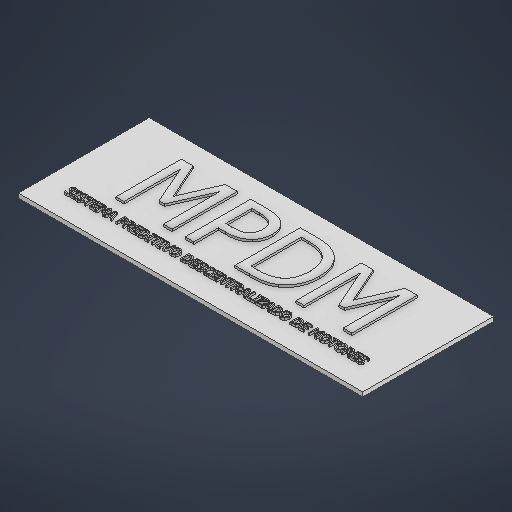
# Autodesk Inventor part: logoR
Saved by Autodesk Inventor 2026.1 (Build 301233020, 233B)
## iProperties
Created: 2025-11-12
Part Number: logoR
Material: Genérico
Document SubType Name: Modeling
Designer: luska
Density: 1 g/cm^3
Appearance: Padrão
Author: luska
## iProperties of the stored document logoR_3DPrint.ipt
Created: 2025-11-12
Part Number: logoR_3DPrint
Material: Genérico
Document SubType Name: Modeling
Designer: luska
Density: 1 g/cm^3
Appearance: Padrão
Author: luska
Autodesk Inventor part; units mm, degrees
ref_plane "YZ Plane" through (0, 0, 0) normal (1, 0, 0) x (0, 1, 0)
ref_plane "XZ Plane" through (0, 0, 0) normal (0, 1, 0) x (-1, 0, 0)
ref_plane "XY Plane" through (0, 0, 0) normal (0, 0, 1) x (1, 0, 0)
sketch "Esboço1" plane through (0, 0, 0) normal (0, 1, 0) x (-1, 0, 0)
  line L0 (65.0365, 6.881) -> (-13.9635, 6.881)
  line L1 (-13.9635, 6.881) -> (-13.9635, -23.119)
  line L2 (-13.9635, -23.119) -> (65.0365, -23.119)
  line L3 (65.0365, -23.119) -> (65.0365, 6.881)
  point P0 (0, 0)
  dimension "d0" = 79
  dimension "d1" = 30
  constraints: 8 end point, 2 parallel, 1 horizontal, 1 perpendicular
  measures "d0" distance between parallel lines of L3 L1
  measures "d1" distance between parallel lines of L2 L0
extrude "Extrusão1" add sketch "Esboço1" along normal blind 1
sketch "Esboço2" plane through (0, 1, 0) normal (0, 1, 0) x (1, 0, 0)
  line L0 (-54.1205, 18.0637) -> (3.0473, 18.0637) construction
  line L1 (3.0473, 18.0637) -> (3.0473, 3.0637) construction
  line L2 (3.0473, 3.0637) -> (-54.1205, 3.0637) construction
  line L3 (-54.1205, 3.0637) -> (-54.1205, 18.0637) construction
  line L4 (-59.7665, 0.1935) -> (8.6922, 0.1935) construction
  line L5 (8.6922, 0.1935) -> (8.6922, -1.8907) construction
  line L6 (8.6922, -1.8907) -> (-59.7665, -1.8907) construction
  line L7 (-59.7665, -1.8907) -> (-59.7665, 0.1935) construction
  line L8 (-65.0365, 23.119) -> (-65.0365, -6.881) projected
  line L9 (13.9635, -6.881) -> (13.9635, 23.119) projected
  line L10 (-39.7404, 3.0637) -> (-41.7339, 3.0637)
  line L11 (-41.7339, 3.0637) -> (-41.7339, 15.9851)
  line L12 (-41.7339, 15.9851) -> (-45.648, 7.1966)
  line L13 (-45.648, 7.1966) -> (-46.8636, 7.1966)
  line L14 (-46.8636, 7.1966) -> (-50.7412, 15.9851)
  line L15 (-50.7412, 15.9851) -> (-50.7412, 3.0637)
  line L16 (-50.7412, 3.0637) -> (-52.601, 3.0637)
  line L17 (-52.601, 3.0637) -> (-52.601, 18.0637)
  line L18 (-52.601, 18.0637) -> (-49.8782, 18.0637)
  line L19 (-49.8782, 18.0637) -> (-46.1342, 9.7128)
  line L20 (-46.1342, 9.7128) -> (-42.5119, 18.0637)
  line L21 (-42.5119, 18.0637) -> (-39.7404, 18.0637)
  line L22 (-39.7404, 18.0637) -> (-39.7404, 3.0637)
  spline S0 degree 2 poles (-27.2201, 13.5418) (-27.2201, 12.5694) (-27.913, 10.819) (-28.5329, 10.2112) knots 0 0 0 1 2 2 2
  spline S1 degree 2 poles (-28.5329, 10.2112) (-29.3109, 9.4454) (-31.4138, 8.6553) (-33.0184, 8.6553) knots 0 0 0 1 2 2 2
  line L23 (-33.0184, 8.6553) -> (-34.708, 8.6553)
  line L24 (-34.708, 8.6553) -> (-34.708, 3.0637)
  line L25 (-34.708, 3.0637) -> (-36.7015, 3.0637)
  line L26 (-36.7015, 3.0637) -> (-36.7015, 18.0637)
  line L27 (-36.7015, 18.0637) -> (-32.9333, 18.0637)
  spline S2 degree 2 poles (-32.9333, 18.0637) (-31.5962, 18.0637) (-29.7242, 17.6261) (-29.007, 17.1277) knots 0 0 0 1 2 2 2
  spline S3 degree 2 poles (-29.007, 17.1277) (-28.1683, 16.5564) (-27.2201, 14.7938) (-27.2201, 13.5418) knots 0 0 0 1 2 2 2
  spline S4 degree 2 poles (-29.2988, 13.481) (-29.2988, 14.259) (-29.8336, 15.4016) (-30.3806, 15.7663) knots 0 0 0 1 2 2 2
  spline S5 degree 2 poles (-30.3806, 15.7663) (-30.8547, 16.0823) (-32.1188, 16.3376) (-33.0548, 16.3376) knots 0 0 0 1 2 2 2
  line L28 (-33.0548, 16.3376) -> (-34.708, 16.3376)
  line L29 (-34.708, 16.3376) -> (-34.708, 10.3571)
  line L30 (-34.708, 10.3571) -> (-33.3466, 10.3571)
  spline S6 degree 2 poles (-33.3466, 10.3571) (-32.131, 10.3571) (-30.6359, 10.746) (-30.1496, 11.2566) knots 0 0 0 1 2 2 2
  spline S7 degree 2 poles (-30.1496, 11.2566) (-29.6999, 11.7063) (-29.2988, 12.7639) (-29.2988, 13.481) knots 0 0 0 1 2 2 2
  spline S8 degree 2 poles (-13.4965, 10.5515) (-13.4965, 8.4972) (-15.1618, 5.1909) (-16.5597, 4.2671) knots 0 0 0 1 2 2 2
  spline S9 degree 2 poles (-16.5597, 4.2671) (-17.7023, 3.5499) (-20.0483, 3.0637) (-21.8717, 3.0637) knots 0 0 0 1 2 2 2
  line L31 (-21.8717, 3.0637) -> (-25.3239, 3.0637)
  line L32 (-25.3239, 3.0637) -> (-25.3239, 18.0637)
  line L33 (-25.3239, 18.0637) -> (-21.9082, 18.0637)
  spline S10 degree 2 poles (-21.9082, 18.0637) (-19.7931, 18.0637) (-17.3863, 17.4316) (-16.5354, 16.8725) knots 0 0 0 1 2 2 2
  spline S11 degree 2 poles (-16.5354, 16.8725) (-15.0889, 15.9122) (-13.4965, 12.7395) (-13.4965, 10.5515) knots 0 0 0 1 2 2 2
  spline S12 degree 2 poles (-15.5751, 10.5759) (-15.5751, 12.3019) (-16.7177, 14.7452) (-17.8482, 15.4381) knots 0 0 0 1 2 2 2
  spline S13 degree 2 poles (-17.8482, 15.4381) (-18.6505, 15.9122) (-20.4616, 16.3376) (-21.8109, 16.3376) knots 0 0 0 1 2 2 2
  line L34 (-21.8109, 16.3376) -> (-23.3304, 16.3376)
  line L35 (-23.3304, 16.3376) -> (-23.3304, 4.7898)
  line L36 (-23.3304, 4.7898) -> (-21.8109, 4.7898)
  spline S14 degree 2 poles (-21.8109, 4.7898) (-20.4859, 4.7898) (-18.4803, 5.2152) (-17.6658, 5.7866) knots 0 0 0 1 2 2 2
  spline S15 degree 2 poles (-17.6658, 5.7866) (-16.6205, 6.4916) (-15.5751, 8.8254) (-15.5751, 10.5759) knots 0 0 0 1 2 2 2
  line L37 (1.5278, 3.0637) -> (-0.4657, 3.0637)
  line L38 (-0.4657, 3.0637) -> (-0.4657, 15.9851)
  line L39 (-0.4657, 15.9851) -> (-4.3798, 7.1966)
  line L40 (-4.3798, 7.1966) -> (-5.5953, 7.1966)
  line L41 (-5.5953, 7.1966) -> (-9.473, 15.9851)
  line L42 (-9.473, 15.9851) -> (-9.473, 3.0637)
  line L43 (-9.473, 3.0637) -> (-11.3328, 3.0637)
  line L44 (-11.3328, 3.0637) -> (-11.3328, 18.0637)
  line L45 (-11.3328, 18.0637) -> (-8.6099, 18.0637)
  line L46 (-8.6099, 18.0637) -> (-4.866, 9.7128)
  line L47 (-4.866, 9.7128) -> (-1.2436, 18.0637)
  line L48 (-1.2436, 18.0637) -> (1.5278, 18.0637)
  line L49 (1.5278, 18.0637) -> (1.5278, 3.0637)
  spline S16 degree 2 poles (-59.0063, -1.8843) (-59.2235, -1.8843) (-59.5282, -1.7935) (-59.6627, -1.7287) knots 0 0 0 1 2 2 2
  line L50 (-59.6627, -1.7287) -> (-59.6627, -1.3948)
  line L51 (-59.6627, -1.3948) -> (-59.6433, -1.3948)
  spline S17 degree 2 poles (-59.6433, -1.3948) (-59.512, -1.518) (-59.1798, -1.6541) (-59.0258, -1.6541) knots 0 0 0 1 2 2 2
  spline S18 degree 2 poles (-59.0258, -1.6541) (-58.8054, -1.6541) (-58.5801, -1.471) (-58.5801, -1.3202) knots 0 0 0 1 2 2 2
  spline S19 degree 2 poles (-58.5801, -1.3202) (-58.5801, -1.2003) (-58.6984, -1.0512) (-58.8264, -1.0139) knots 0 0 0 1 2 2 2
  spline S20 degree 2 poles (-58.8264, -1.0139) (-58.9188, -0.988) (-59.0728, -0.9523) (-59.1879, -0.9232) knots 0 0 0 1 2 2 2
  spline S21 degree 2 poles (-59.1879, -0.9232) (-59.2916, -0.8956) (-59.4553, -0.8129) (-59.5185, -0.7465) knots 0 0 0 1 2 2 2
  spline S22 degree 2 poles (-59.5185, -0.7465) (-59.5801, -0.68) (-59.6482, -0.5018) (-59.6482, -0.3851) knots 0 0 0 1 2 2 2
  spline S23 degree 2 poles (-59.6482, -0.3851) (-59.6482, -0.142) (-59.2689, 0.1871) (-58.9755, 0.1871) knots 0 0 0 1 2 2 2
  spline S24 degree 2 poles (-58.9755, 0.1871) (-58.807, 0.1871) (-58.5088, 0.1206) (-58.3807, 0.0574) knots 0 0 0 1 2 2 2
  line L52 (-58.3807, 0.0574) -> (-58.3807, -0.2603)
  line L53 (-58.3807, -0.2603) -> (-58.4002, -0.2603)
  spline S25 degree 2 poles (-58.4002, -0.2603) (-58.4958, -0.1728) (-58.794, -0.0431) (-58.9577, -0.0431) knots 0 0 0 1 2 2 2
  spline S26 degree 2 poles (-58.9577, -0.0431) (-59.1425, -0.0431) (-59.371, -0.2165) (-59.371, -0.3575) knots 0 0 0 1 2 2 2
  spline S27 degree 2 poles (-59.371, -0.3575) (-59.371, -0.4839) (-59.2365, -0.6347) (-59.1101, -0.6687) knots 0 0 0 1 2 2 2
  spline S28 degree 2 poles (-59.1101, -0.6687) (-59.0258, -0.6914) (-58.7811, -0.7497) (-58.7, -0.774) knots 0 0 0 1 2 2 2
  spline S29 degree 2 poles (-58.7, -0.774) (-58.4942, -0.8373) (-58.3029, -1.0917) (-58.3029, -1.2781) knots 0 0 0 1 2 2 2
  spline S30 degree 2 poles (-58.3029, -1.2781) (-58.3029, -1.3964) (-58.3986, -1.6233) (-58.4845, -1.7027) knots 0 0 0 1 2 2 2
  spline S31 degree 2 poles (-58.4845, -1.7027) (-58.5801, -1.7903) (-58.8232, -1.8843) (-59.0063, -1.8843) knots 0 0 0 1 2 2 2
  line L54 (-57.3353, -1.8486) -> (-58.1101, -1.8486)
  line L55 (-58.1101, -1.8486) -> (-58.1101, -1.6444)
  line L56 (-58.1101, -1.6444) -> (-57.8556, -1.6444)
  line L57 (-57.8556, -1.6444) -> (-57.8556, -0.0528)
  line L58 (-57.8556, -0.0528) -> (-58.1101, -0.0528)
  line L59 (-58.1101, -0.0528) -> (-58.1101, 0.1514)
  line L60 (-58.1101, 0.1514) -> (-57.3353, 0.1514)
  line L61 (-57.3353, 0.1514) -> (-57.3353, -0.0528)
  line L62 (-57.3353, -0.0528) -> (-57.5898, -0.0528)
  line L63 (-57.5898, -0.0528) -> (-57.5898, -1.6444)
  line L64 (-57.5898, -1.6444) -> (-57.3353, -1.6444)
  line L65 (-57.3353, -1.6444) -> (-57.3353, -1.8486)
  spline S32 degree 2 poles (-56.4488, -1.8843) (-56.666, -1.8843) (-56.9707, -1.7935) (-57.1052, -1.7287) knots 0 0 0 1 2 2 2
  line L66 (-57.1052, -1.7287) -> (-57.1052, -1.3948)
  line L67 (-57.1052, -1.3948) -> (-57.0858, -1.3948)
  spline S33 degree 2 poles (-57.0858, -1.3948) (-56.9545, -1.518) (-56.6222, -1.6541) (-56.4683, -1.6541) knots 0 0 0 1 2 2 2
  spline S34 degree 2 poles (-56.4683, -1.6541) (-56.2478, -1.6541) (-56.0225, -1.471) (-56.0225, -1.3202) knots 0 0 0 1 2 2 2
  spline S35 degree 2 poles (-56.0225, -1.3202) (-56.0225, -1.2003) (-56.1409, -1.0512) (-56.2689, -1.0139) knots 0 0 0 1 2 2 2
  spline S36 degree 2 poles (-56.2689, -1.0139) (-56.3613, -0.988) (-56.5153, -0.9523) (-56.6303, -0.9232) knots 0 0 0 1 2 2 2
  spline S37 degree 2 poles (-56.6303, -0.9232) (-56.7341, -0.8956) (-56.8977, -0.8129) (-56.961, -0.7465) knots 0 0 0 1 2 2 2
  spline S38 degree 2 poles (-56.961, -0.7465) (-57.0225, -0.68) (-57.0906, -0.5018) (-57.0906, -0.3851) knots 0 0 0 1 2 2 2
  spline S39 degree 2 poles (-57.0906, -0.3851) (-57.0906, -0.142) (-56.7114, 0.1871) (-56.418, 0.1871) knots 0 0 0 1 2 2 2
  spline S40 degree 2 poles (-56.418, 0.1871) (-56.2495, 0.1871) (-55.9512, 0.1206) (-55.8232, 0.0574) knots 0 0 0 1 2 2 2
  line L68 (-55.8232, 0.0574) -> (-55.8232, -0.2603)
  line L69 (-55.8232, -0.2603) -> (-55.8426, -0.2603)
  spline S41 degree 2 poles (-55.8426, -0.2603) (-55.9383, -0.1728) (-56.2365, -0.0431) (-56.4002, -0.0431) knots 0 0 0 1 2 2 2
  spline S42 degree 2 poles (-56.4002, -0.0431) (-56.5849, -0.0431) (-56.8135, -0.2165) (-56.8135, -0.3575) knots 0 0 0 1 2 2 2
  spline S43 degree 2 poles (-56.8135, -0.3575) (-56.8135, -0.4839) (-56.6789, -0.6347) (-56.5525, -0.6687) knots 0 0 0 1 2 2 2
  spline S44 degree 2 poles (-56.5525, -0.6687) (-56.4683, -0.6914) (-56.2235, -0.7497) (-56.1425, -0.774) knots 0 0 0 1 2 2 2
  spline S45 degree 2 poles (-56.1425, -0.774) (-55.9366, -0.8373) (-55.7454, -1.0917) (-55.7454, -1.2781) knots 0 0 0 1 2 2 2
  spline S46 degree 2 poles (-55.7454, -1.2781) (-55.7454, -1.3964) (-55.841, -1.6233) (-55.9269, -1.7027) knots 0 0 0 1 2 2 2
  spline S47 degree 2 poles (-55.9269, -1.7027) (-56.0225, -1.7903) (-56.2657, -1.8843) (-56.4488, -1.8843) knots 0 0 0 1 2 2 2
  line L70 (-55.008, -1.8486) -> (-55.008, -0.0852)
  line L71 (-55.008, -0.0852) -> (-55.6789, -0.0852)
  line L72 (-55.6789, -0.0852) -> (-55.6789, 0.1514)
  line L73 (-55.6789, 0.1514) -> (-54.0712, 0.1514)
  line L74 (-54.0712, 0.1514) -> (-54.0712, -0.0852)
  line L75 (-54.0712, -0.0852) -> (-54.7422, -0.0852)
  line L76 (-54.7422, -0.0852) -> (-54.7422, -1.8486)
  line L77 (-54.7422, -1.8486) -> (-55.008, -1.8486)
  line L78 (-53.8686, -1.8486) -> (-53.8686, 0.1514)
  line L79 (-53.8686, 0.1514) -> (-52.6174, 0.1514)
  line L80 (-52.6174, 0.1514) -> (-52.6174, -0.0852)
  line L81 (-52.6174, -0.0852) -> (-53.6028, -0.0852)
  line L82 (-53.6028, -0.0852) -> (-53.6028, -0.633)
  line L83 (-53.6028, -0.633) -> (-52.6838, -0.633)
  line L84 (-52.6838, -0.633) -> (-52.6838, -0.8697)
  line L85 (-52.6838, -0.8697) -> (-53.6028, -0.8697)
  line L86 (-53.6028, -0.8697) -> (-53.6028, -1.612)
  line L87 (-53.6028, -1.612) -> (-52.6174, -1.612)
  line L88 (-52.6174, -1.612) -> (-52.6174, -1.8486)
  line L89 (-52.6174, -1.8486) -> (-53.8686, -1.8486)
  line L90 (-50.6109, -1.8486) -> (-50.8767, -1.8486)
  line L91 (-50.8767, -1.8486) -> (-50.8767, -0.1258)
  line L92 (-50.8767, -0.1258) -> (-51.3986, -1.2976)
  line L93 (-51.3986, -1.2976) -> (-51.5606, -1.2976)
  line L94 (-51.5606, -1.2976) -> (-52.0777, -0.1258)
  line L95 (-52.0777, -0.1258) -> (-52.0777, -1.8486)
  line L96 (-52.0777, -1.8486) -> (-52.3256, -1.8486)
  line L97 (-52.3256, -1.8486) -> (-52.3256, 0.1514)
  line L98 (-52.3256, 0.1514) -> (-51.9626, 0.1514)
  line L99 (-51.9626, 0.1514) -> (-51.4634, -0.9621)
  line L100 (-51.4634, -0.9621) -> (-50.9804, 0.1514)
  line L101 (-50.9804, 0.1514) -> (-50.6109, 0.1514)
  line L102 (-50.6109, 0.1514) -> (-50.6109, -1.8486)
  line L103 (-50.4212, -1.8486) -> (-49.747, 0.1514)
  line L104 (-49.747, 0.1514) -> (-49.4196, 0.1514)
  line L105 (-49.4196, 0.1514) -> (-48.7454, -1.8486)
  line L106 (-48.7454, -1.8486) -> (-49.0258, -1.8486)
  line L107 (-49.0258, -1.8486) -> (-49.2073, -1.2894)
  line L108 (-49.2073, -1.2894) -> (-49.9707, -1.2894)
  line L109 (-49.9707, -1.2894) -> (-50.1522, -1.8486)
  line L110 (-50.1522, -1.8486) -> (-50.4212, -1.8486)
  line L111 (-49.2802, -1.0625) -> (-49.5898, -0.1209)
  line L112 (-49.5898, -0.1209) -> (-49.8977, -1.0625)
  line L113 (-49.8977, -1.0625) -> (-49.2802, -1.0625)
  spline S48 degree 2 poles (-46.4326, -0.4515) (-46.4326, -0.5812) (-46.525, -0.8146) (-46.6076, -0.8956) knots 0 0 0 1 2 2 2
  spline S49 degree 2 poles (-46.6076, -0.8956) (-46.7114, -0.9977) (-46.9918, -1.1031) (-47.2057, -1.1031) knots 0 0 0 1 2 2 2
  line L114 (-47.2057, -1.1031) -> (-47.431, -1.1031)
  line L115 (-47.431, -1.1031) -> (-47.431, -1.8486)
  line L116 (-47.431, -1.8486) -> (-47.6968, -1.8486)
  line L117 (-47.6968, -1.8486) -> (-47.6968, 0.1514)
  line L118 (-47.6968, 0.1514) -> (-47.1943, 0.1514)
  spline S50 degree 2 poles (-47.1943, 0.1514) (-47.0161, 0.1514) (-46.7665, 0.093) (-46.6708, 0.0266) knots 0 0 0 1 2 2 2
  spline S51 degree 2 poles (-46.6708, 0.0266) (-46.559, -0.0496) (-46.4326, -0.2846) (-46.4326, -0.4515) knots 0 0 0 1 2 2 2
  spline S52 degree 2 poles (-46.7097, -0.4596) (-46.7097, -0.3559) (-46.7811, -0.2035) (-46.854, -0.1549) knots 0 0 0 1 2 2 2
  spline S53 degree 2 poles (-46.854, -0.1549) (-46.9172, -0.1128) (-47.0858, -0.0787) (-47.2106, -0.0787) knots 0 0 0 1 2 2 2
  line L119 (-47.2106, -0.0787) -> (-47.431, -0.0787)
  line L120 (-47.431, -0.0787) -> (-47.431, -0.8762)
  line L121 (-47.431, -0.8762) -> (-47.2495, -0.8762)
  spline S54 degree 2 poles (-47.2495, -0.8762) (-47.0874, -0.8762) (-46.888, -0.8243) (-46.8232, -0.7562) knots 0 0 0 1 2 2 2
  spline S55 degree 2 poles (-46.8232, -0.7562) (-46.7632, -0.6963) (-46.7097, -0.5552) (-46.7097, -0.4596) knots 0 0 0 1 2 2 2
  line L122 (-44.6319, -1.8486) -> (-44.9772, -1.8486)
  line L123 (-44.9772, -1.8486) -> (-45.6093, -1.0528)
  line L124 (-45.6093, -1.0528) -> (-45.914, -1.0528)
  line L125 (-45.914, -1.0528) -> (-45.914, -1.8486)
  line L126 (-45.914, -1.8486) -> (-46.1798, -1.8486)
  line L127 (-46.1798, -1.8486) -> (-46.1798, 0.1514)
  line L128 (-46.1798, 0.1514) -> (-45.6644, 0.1514)
  spline S56 degree 2 poles (-45.6644, 0.1514) (-45.4926, 0.1514) (-45.2608, 0.1141) (-45.1554, 0.046) knots 0 0 0 1 2 2 2
  spline S57 degree 2 poles (-45.1554, 0.046) (-45.0501, -0.022) (-44.9285, -0.2343) (-44.9285, -0.3916) knots 0 0 0 1 2 2 2
  spline S58 degree 2 poles (-44.9285, -0.3916) (-44.9285, -0.6104) (-45.1522, -0.907) (-45.3435, -0.9783) knots 0 0 0 1 2 2 2
  line L129 (-45.3435, -0.9783) -> (-44.6319, -1.8486)
  spline S59 degree 2 poles (-45.2057, -0.4126) (-45.2057, -0.3251) (-45.2673, -0.1906) (-45.3321, -0.1468) knots 0 0 0 1 2 2 2
  spline S60 degree 2 poles (-45.3321, -0.1468) (-45.3888, -0.1095) (-45.5396, -0.0787) (-45.6498, -0.0787) knots 0 0 0 1 2 2 2
  line L130 (-45.6498, -0.0787) -> (-45.914, -0.0787)
  line L131 (-45.914, -0.0787) -> (-45.914, -0.8308)
  line L132 (-45.914, -0.8308) -> (-45.6806, -0.8308)
  spline S61 degree 2 poles (-45.6806, -0.8308) (-45.5655, -0.8308) (-45.3824, -0.7903) (-45.3191, -0.727) knots 0 0 0 1 2 2 2
  spline S62 degree 2 poles (-45.3191, -0.727) (-45.2608, -0.6719) (-45.2057, -0.5164) (-45.2057, -0.4126) knots 0 0 0 1 2 2 2
  line L133 (-44.4731, -1.8486) -> (-44.4731, 0.1514)
  line L134 (-44.4731, 0.1514) -> (-43.2219, 0.1514)
  line L135 (-43.2219, 0.1514) -> (-43.2219, -0.0852)
  line L136 (-43.2219, -0.0852) -> (-44.2073, -0.0852)
  line L137 (-44.2073, -0.0852) -> (-44.2073, -0.633)
  line L138 (-44.2073, -0.633) -> (-43.2883, -0.633)
  line L139 (-43.2883, -0.633) -> (-43.2883, -0.8697)
  line L140 (-43.2883, -0.8697) -> (-44.2073, -0.8697)
  line L141 (-44.2073, -0.8697) -> (-44.2073, -1.612)
  line L142 (-44.2073, -1.612) -> (-43.2219, -1.612)
  line L143 (-43.2219, -1.612) -> (-43.2219, -1.8486)
  line L144 (-43.2219, -1.8486) -> (-44.4731, -1.8486)
  spline S63 degree 2 poles (-41.3532, -0.8502) (-41.3532, -1.1241) (-41.5752, -1.565) (-41.7616, -1.6881) knots 0 0 0 1 2 2 2
  spline S64 degree 2 poles (-41.7616, -1.6881) (-41.914, -1.7838) (-42.2268, -1.8486) (-42.4699, -1.8486) knots 0 0 0 1 2 2 2
  line L145 (-42.4699, -1.8486) -> (-42.9302, -1.8486)
  line L146 (-42.9302, -1.8486) -> (-42.9302, 0.1514)
  line L147 (-42.9302, 0.1514) -> (-42.4747, 0.1514)
  spline S65 degree 2 poles (-42.4747, 0.1514) (-42.1927, 0.1514) (-41.8718, 0.0671) (-41.7584, -0.0074) knots 0 0 0 1 2 2 2
  spline S66 degree 2 poles (-41.7584, -0.0074) (-41.5655, -0.1355) (-41.3532, -0.5585) (-41.3532, -0.8502) knots 0 0 0 1 2 2 2
  spline S67 degree 2 poles (-41.6303, -0.847) (-41.6303, -0.6168) (-41.7827, -0.2911) (-41.9334, -0.1987) knots 0 0 0 1 2 2 2
  spline S68 degree 2 poles (-41.9334, -0.1987) (-42.0404, -0.1355) (-42.2819, -0.0787) (-42.4618, -0.0787) knots 0 0 0 1 2 2 2
  line L148 (-42.4618, -0.0787) -> (-42.6644, -0.0787)
  line L149 (-42.6644, -0.0787) -> (-42.6644, -1.6185)
  line L150 (-42.6644, -1.6185) -> (-42.4618, -1.6185)
  spline S69 degree 2 poles (-42.4618, -1.6185) (-42.2851, -1.6185) (-42.0177, -1.5617) (-41.9091, -1.4856) knots 0 0 0 1 2 2 2
  spline S70 degree 2 poles (-41.9091, -1.4856) (-41.7697, -1.3916) (-41.6303, -1.0804) (-41.6303, -0.847) knots 0 0 0 1 2 2 2
  line L151 (-40.3678, -1.8486) -> (-41.1425, -1.8486)
  line L152 (-41.1425, -1.8486) -> (-41.1425, -1.6444)
  line L153 (-41.1425, -1.6444) -> (-40.888, -1.6444)
  line L154 (-40.888, -1.6444) -> (-40.888, -0.0528)
  line L155 (-40.888, -0.0528) -> (-41.1425, -0.0528)
  line L156 (-41.1425, -0.0528) -> (-41.1425, 0.1514)
  line L157 (-41.1425, 0.1514) -> (-40.3678, 0.1514)
  line L158 (-40.3678, 0.1514) -> (-40.3678, -0.0528)
  line L159 (-40.3678, -0.0528) -> (-40.6222, -0.0528)
  line L160 (-40.6222, -0.0528) -> (-40.6222, -1.6444)
  line L161 (-40.6222, -1.6444) -> (-40.3678, -1.6444)
  line L162 (-40.3678, -1.6444) -> (-40.3678, -1.8486)
  line L163 (-39.572, -1.8486) -> (-39.572, -0.0852)
  line L164 (-39.572, -0.0852) -> (-40.243, -0.0852)
  line L165 (-40.243, -0.0852) -> (-40.243, 0.1514)
  line L166 (-40.243, 0.1514) -> (-38.6352, 0.1514)
  line L167 (-38.6352, 0.1514) -> (-38.6352, -0.0852)
  line L168 (-38.6352, -0.0852) -> (-39.3062, -0.0852)
  line L169 (-39.3062, -0.0852) -> (-39.3062, -1.8486)
  line L170 (-39.3062, -1.8486) -> (-39.572, -1.8486)
  line L171 (-37.7357, -1.8486) -> (-38.5104, -1.8486)
  line L172 (-38.5104, -1.8486) -> (-38.5104, -1.6444)
  line L173 (-38.5104, -1.6444) -> (-38.2559, -1.6444)
  line L174 (-38.2559, -1.6444) -> (-38.2559, -0.0528)
  line L175 (-38.2559, -0.0528) -> (-38.5104, -0.0528)
  line L176 (-38.5104, -0.0528) -> (-38.5104, 0.1514)
  line L177 (-38.5104, 0.1514) -> (-37.7357, 0.1514)
  line L178 (-37.7357, 0.1514) -> (-37.7357, -0.0528)
  line L179 (-37.7357, -0.0528) -> (-37.9901, -0.0528)
  line L180 (-37.9901, -0.0528) -> (-37.9901, -1.6444)
  line L181 (-37.9901, -1.6444) -> (-37.7357, -1.6444)
  line L182 (-37.7357, -1.6444) -> (-37.7357, -1.8486)
  line L183 (-35.9561, 0.1514) -> (-36.6449, -1.8486)
  line L184 (-36.6449, -1.8486) -> (-36.9318, -1.8486)
  line L185 (-36.9318, -1.8486) -> (-37.6206, 0.1514)
  line L186 (-37.6206, 0.1514) -> (-37.3353, 0.1514)
  line L187 (-37.3353, 0.1514) -> (-36.7811, -1.5099)
  line L188 (-36.7811, -1.5099) -> (-36.2268, 0.1514)
  line L189 (-36.2268, 0.1514) -> (-35.9561, 0.1514)
  spline S71 degree 2 poles (-34.3499, -0.0771) (-34.2365, -0.21) (-34.1101, -0.599) (-34.1101, -0.8486) knots 0 0 0 1 2 2 2
  spline S72 degree 2 poles (-34.1101, -0.8486) (-34.1101, -1.0917) (-34.2332, -1.4856) (-34.3499, -1.6185) knots 0 0 0 1 2 2 2
  spline S73 degree 2 poles (-34.3499, -1.6185) (-34.4731, -1.7578) (-34.7989, -1.8907) (-34.995, -1.8907) knots 0 0 0 1 2 2 2
  spline S74 degree 2 poles (-34.995, -1.8907) (-35.1976, -1.8907) (-35.5217, -1.753) (-35.64, -1.6185) knots 0 0 0 1 2 2 2
  spline S75 degree 2 poles (-35.64, -1.6185) (-35.7551, -1.4856) (-35.8783, -1.095) (-35.8783, -0.8486) knots 0 0 0 1 2 2 2
  spline S76 degree 2 poles (-35.8783, -0.8486) (-35.8783, -0.5974) (-35.7535, -0.2149) (-35.6384, -0.0771) knots 0 0 0 1 2 2 2
  spline S77 degree 2 poles (-35.6384, -0.0771) (-35.5217, 0.0558) (-35.196, 0.1935) (-34.995, 0.1935) knots 0 0 0 1 2 2 2
  spline S78 degree 2 poles (-34.995, 0.1935) (-34.7908, 0.1935) (-34.4634, 0.0509) (-34.3499, -0.0771) knots 0 0 0 1 2 2 2
  spline S79 degree 2 poles (-34.3872, -0.8486) (-34.3872, -0.6509) (-34.4731, -0.3446) (-34.5509, -0.2441) knots 0 0 0 1 2 2 2
  spline S80 degree 2 poles (-34.5509, -0.2441) (-34.6303, -0.1403) (-34.854, -0.0366) (-34.9934, -0.0366) knots 0 0 0 1 2 2 2
  spline S81 degree 2 poles (-34.9934, -0.0366) (-35.1376, -0.0366) (-35.3548, -0.1371) (-35.4375, -0.2441) knots 0 0 0 1 2 2 2
  spline S82 degree 2 poles (-35.4375, -0.2441) (-35.5169, -0.3462) (-35.6012, -0.6541) (-35.6012, -0.8486) knots 0 0 0 1 2 2 2
  spline S83 degree 2 poles (-35.6012, -0.8486) (-35.6012, -1.2424) (-35.2705, -1.6606) (-34.9934, -1.6606) knots 0 0 0 1 2 2 2
  spline S84 degree 2 poles (-34.9934, -1.6606) (-34.7162, -1.6606) (-34.3872, -1.2424) (-34.3872, -0.8486) knots 0 0 0 1 2 2 2
  spline S85 degree 2 poles (-31.3824, -0.8502) (-31.3824, -1.1241) (-31.6044, -1.565) (-31.7908, -1.6881) knots 0 0 0 1 2 2 2
  spline S86 degree 2 poles (-31.7908, -1.6881) (-31.9431, -1.7838) (-32.2559, -1.8486) (-32.499, -1.8486) knots 0 0 0 1 2 2 2
  line L190 (-32.499, -1.8486) -> (-32.9593, -1.8486)
  line L191 (-32.9593, -1.8486) -> (-32.9593, 0.1514)
  line L192 (-32.9593, 0.1514) -> (-32.5039, 0.1514)
  spline S87 degree 2 poles (-32.5039, 0.1514) (-32.2219, 0.1514) (-31.901, 0.0671) (-31.7875, -0.0074) knots 0 0 0 1 2 2 2
  spline S88 degree 2 poles (-31.7875, -0.0074) (-31.5947, -0.1355) (-31.3824, -0.5585) (-31.3824, -0.8502) knots 0 0 0 1 2 2 2
  spline S89 degree 2 poles (-31.6595, -0.847) (-31.6595, -0.6168) (-31.8118, -0.2911) (-31.9626, -0.1987) knots 0 0 0 1 2 2 2
  spline S90 degree 2 poles (-31.9626, -0.1987) (-32.0695, -0.1355) (-32.311, -0.0787) (-32.4909, -0.0787) knots 0 0 0 1 2 2 2
  line L193 (-32.4909, -0.0787) -> (-32.6935, -0.0787)
  line L194 (-32.6935, -0.0787) -> (-32.6935, -1.6185)
  line L195 (-32.6935, -1.6185) -> (-32.4909, -1.6185)
  spline S91 degree 2 poles (-32.4909, -1.6185) (-32.3143, -1.6185) (-32.0469, -1.5617) (-31.9383, -1.4856) knots 0 0 0 1 2 2 2
  spline S92 degree 2 poles (-31.9383, -1.4856) (-31.7989, -1.3916) (-31.6595, -1.0804) (-31.6595, -0.847) knots 0 0 0 1 2 2 2
  line L196 (-31.0939, -1.8486) -> (-31.0939, 0.1514)
  line L197 (-31.0939, 0.1514) -> (-29.8426, 0.1514)
  line L198 (-29.8426, 0.1514) -> (-29.8426, -0.0852)
  line L199 (-29.8426, -0.0852) -> (-30.8281, -0.0852)
  line L200 (-30.8281, -0.0852) -> (-30.8281, -0.633)
  line L201 (-30.8281, -0.633) -> (-29.9091, -0.633)
  line L202 (-29.9091, -0.633) -> (-29.9091, -0.8697)
  line L203 (-29.9091, -0.8697) -> (-30.8281, -0.8697)
  line L204 (-30.8281, -0.8697) -> (-30.8281, -1.612)
  line L205 (-30.8281, -1.612) -> (-29.8426, -1.612)
  line L206 (-29.8426, -1.612) -> (-29.8426, -1.8486)
  line L207 (-29.8426, -1.8486) -> (-31.0939, -1.8486)
  spline S93 degree 2 poles (-28.9934, -1.8843) (-29.2106, -1.8843) (-29.5153, -1.7935) (-29.6498, -1.7287) knots 0 0 0 1 2 2 2
  line L208 (-29.6498, -1.7287) -> (-29.6498, -1.3948)
  line L209 (-29.6498, -1.3948) -> (-29.6303, -1.3948)
  spline S94 degree 2 poles (-29.6303, -1.3948) (-29.499, -1.518) (-29.1668, -1.6541) (-29.0128, -1.6541) knots 0 0 0 1 2 2 2
  spline S95 degree 2 poles (-29.0128, -1.6541) (-28.7924, -1.6541) (-28.5671, -1.471) (-28.5671, -1.3202) knots 0 0 0 1 2 2 2
  spline S96 degree 2 poles (-28.5671, -1.3202) (-28.5671, -1.2003) (-28.6854, -1.0512) (-28.8135, -1.0139) knots 0 0 0 1 2 2 2
  spline S97 degree 2 poles (-28.8135, -1.0139) (-28.9059, -0.988) (-29.0598, -0.9523) (-29.1749, -0.9232) knots 0 0 0 1 2 2 2
  spline S98 degree 2 poles (-29.1749, -0.9232) (-29.2786, -0.8956) (-29.4423, -0.8129) (-29.5055, -0.7465) knots 0 0 0 1 2 2 2
  spline S99 degree 2 poles (-29.5055, -0.7465) (-29.5671, -0.68) (-29.6352, -0.5018) (-29.6352, -0.3851) knots 0 0 0 1 2 2 2
  spline S100 degree 2 poles (-29.6352, -0.3851) (-29.6352, -0.142) (-29.2559, 0.1871) (-28.9626, 0.1871) knots 0 0 0 1 2 2 2
  spline S101 degree 2 poles (-28.9626, 0.1871) (-28.794, 0.1871) (-28.4958, 0.1206) (-28.3678, 0.0574) knots 0 0 0 1 2 2 2
  line L210 (-28.3678, 0.0574) -> (-28.3678, -0.2603)
  line L211 (-28.3678, -0.2603) -> (-28.3872, -0.2603)
  spline S102 degree 2 poles (-28.3872, -0.2603) (-28.4828, -0.1728) (-28.7811, -0.0431) (-28.9447, -0.0431) knots 0 0 0 1 2 2 2
  spline S103 degree 2 poles (-28.9447, -0.0431) (-29.1295, -0.0431) (-29.358, -0.2165) (-29.358, -0.3575) knots 0 0 0 1 2 2 2
  spline S104 degree 2 poles (-29.358, -0.3575) (-29.358, -0.4839) (-29.2235, -0.6347) (-29.0971, -0.6687) knots 0 0 0 1 2 2 2
  spline S105 degree 2 poles (-29.0971, -0.6687) (-29.0128, -0.6914) (-28.7681, -0.7497) (-28.6871, -0.774) knots 0 0 0 1 2 2 2
  spline S106 degree 2 poles (-28.6871, -0.774) (-28.4812, -0.8373) (-28.29, -1.0917) (-28.29, -1.2781) knots 0 0 0 1 2 2 2
  spline S107 degree 2 poles (-28.29, -1.2781) (-28.29, -1.3964) (-28.3856, -1.6233) (-28.4715, -1.7027) knots 0 0 0 1 2 2 2
  spline S108 degree 2 poles (-28.4715, -1.7027) (-28.5671, -1.7903) (-28.8102, -1.8843) (-28.9934, -1.8843) knots 0 0 0 1 2 2 2
  spline S109 degree 2 poles (-27.2381, -1.8843) (-27.4326, -1.8843) (-27.7616, -1.753) (-27.8815, -1.6217) knots 0 0 0 1 2 2 2
  spline S110 degree 2 poles (-27.8815, -1.6217) (-28.0015, -1.492) (-28.1328, -1.1031) (-28.1328, -0.8502) knots 0 0 0 1 2 2 2
  spline S111 degree 2 poles (-28.1328, -0.8502) (-28.1328, -0.599) (-28.0047, -0.2262) (-27.8832, -0.0885) knots 0 0 0 1 2 2 2
  spline S112 degree 2 poles (-27.8832, -0.0885) (-27.7632, 0.046) (-27.4358, 0.1871) (-27.2332, 0.1871) knots 0 0 0 1 2 2 2
  spline S113 degree 2 poles (-27.2332, 0.1871) (-27.1328, 0.1871) (-26.9561, 0.1579) (-26.8815, 0.1352) knots 0 0 0 1 2 2 2
  spline S114 degree 2 poles (-26.8815, 0.1352) (-26.8167, 0.1141) (-26.6822, 0.0542) (-26.6157, 0.0185) knots 0 0 0 1 2 2 2
  line L212 (-26.6157, 0.0185) -> (-26.6157, -0.3024)
  line L213 (-26.6157, -0.3024) -> (-26.6368, -0.3024)
  spline S115 degree 2 poles (-26.6368, -0.3024) (-26.6725, -0.27) (-26.7827, -0.1792) (-26.8621, -0.1355) knots 0 0 0 1 2 2 2
  spline S116 degree 2 poles (-26.8621, -0.1355) (-26.9383, -0.0933) (-27.1182, -0.0399) (-27.2349, -0.0399) knots 0 0 0 1 2 2 2
  spline S117 degree 2 poles (-27.2349, -0.0399) (-27.3629, -0.0399) (-27.5914, -0.1452) (-27.6773, -0.2457) knots 0 0 0 1 2 2 2
  spline S118 degree 2 poles (-27.6773, -0.2457) (-27.7616, -0.3478) (-27.8556, -0.6574) (-27.8556, -0.8502) knots 0 0 0 1 2 2 2
  spline S119 degree 2 poles (-27.8556, -0.8502) (-27.8556, -1.0561) (-27.7567, -1.3527) (-27.6708, -1.4548) knots 0 0 0 1 2 2 2
  spline S120 degree 2 poles (-27.6708, -1.4548) (-27.5866, -1.5536) (-27.3613, -1.6541) (-27.2349, -1.6541) knots 0 0 0 1 2 2 2
  spline S121 degree 2 poles (-27.2349, -1.6541) (-27.1198, -1.6541) (-26.9237, -1.5974) (-26.8475, -1.5552) knots 0 0 0 1 2 2 2
  spline S122 degree 2 poles (-26.8475, -1.5552) (-26.7746, -1.5131) (-26.666, -1.4256) (-26.6352, -1.3948) knots 0 0 0 1 2 2 2
  line L214 (-26.6352, -1.3948) -> (-26.6157, -1.3948)
  line L215 (-26.6157, -1.3948) -> (-26.6157, -1.7125)
  spline S123 degree 2 poles (-26.6157, -1.7125) (-26.6822, -1.7433) (-26.7989, -1.8) (-26.8815, -1.8259) knots 0 0 0 1 2 2 2
  spline S124 degree 2 poles (-26.8815, -1.8259) (-26.9691, -1.8551) (-27.1182, -1.8843) (-27.2381, -1.8843) knots 0 0 0 1 2 2 2
  line L216 (-26.3678, -1.8486) -> (-26.3678, 0.1514)
  line L217 (-26.3678, 0.1514) -> (-25.1165, 0.1514)
  line L218 (-25.1165, 0.1514) -> (-25.1165, -0.0852)
  line L219 (-25.1165, -0.0852) -> (-26.102, -0.0852)
  line L220 (-26.102, -0.0852) -> (-26.102, -0.633)
  line L221 (-26.102, -0.633) -> (-25.183, -0.633)
  line L222 (-25.183, -0.633) -> (-25.183, -0.8697)
  line L223 (-25.183, -0.8697) -> (-26.102, -0.8697)
  line L224 (-26.102, -0.8697) -> (-26.102, -1.612)
  line L225 (-26.102, -1.612) -> (-25.1165, -1.612)
  line L226 (-25.1165, -1.612) -> (-25.1165, -1.8486)
  line L227 (-25.1165, -1.8486) -> (-26.3678, -1.8486)
  line L228 (-23.3937, -1.8486) -> (-23.6919, -1.8486)
  line L229 (-23.6919, -1.8486) -> (-24.5768, -0.1241)
  line L230 (-24.5768, -0.1241) -> (-24.5768, -1.8486)
  line L231 (-24.5768, -1.8486) -> (-24.8248, -1.8486)
  line L232 (-24.8248, -1.8486) -> (-24.8248, 0.1514)
  line L233 (-24.8248, 0.1514) -> (-24.4472, 0.1514)
  line L234 (-24.4472, 0.1514) -> (-23.6417, -1.4321)
  line L235 (-23.6417, -1.4321) -> (-23.6417, 0.1514)
  line L236 (-23.6417, 0.1514) -> (-23.3937, 0.1514)
  line L237 (-23.3937, 0.1514) -> (-23.3937, -1.8486)
  line L238 (-22.5217, -1.8486) -> (-22.5217, -0.0852)
  line L239 (-22.5217, -0.0852) -> (-23.1927, -0.0852)
  line L240 (-23.1927, -0.0852) -> (-23.1927, 0.1514)
  line L241 (-23.1927, 0.1514) -> (-21.5849, 0.1514)
  line L242 (-21.5849, 0.1514) -> (-21.5849, -0.0852)
  line L243 (-21.5849, -0.0852) -> (-22.2559, -0.0852)
  line L244 (-22.2559, -0.0852) -> (-22.2559, -1.8486)
  line L245 (-22.2559, -1.8486) -> (-22.5217, -1.8486)
  line L246 (-19.8345, -1.8486) -> (-20.1798, -1.8486)
  line L247 (-20.1798, -1.8486) -> (-20.8118, -1.0528)
  line L248 (-20.8118, -1.0528) -> (-21.1165, -1.0528)
  line L249 (-21.1165, -1.0528) -> (-21.1165, -1.8486)
  line L250 (-21.1165, -1.8486) -> (-21.3824, -1.8486)
  line L251 (-21.3824, -1.8486) -> (-21.3824, 0.1514)
  line L252 (-21.3824, 0.1514) -> (-20.867, 0.1514)
  spline S125 degree 2 poles (-20.867, 0.1514) (-20.6952, 0.1514) (-20.4634, 0.1141) (-20.358, 0.046) knots 0 0 0 1 2 2 2
  spline S126 degree 2 poles (-20.358, 0.046) (-20.2527, -0.022) (-20.1311, -0.2343) (-20.1311, -0.3916) knots 0 0 0 1 2 2 2
  spline S127 degree 2 poles (-20.1311, -0.3916) (-20.1311, -0.6104) (-20.3548, -0.907) (-20.546, -0.9783) knots 0 0 0 1 2 2 2
  line L253 (-20.546, -0.9783) -> (-19.8345, -1.8486)
  spline S128 degree 2 poles (-20.4083, -0.4126) (-20.4083, -0.3251) (-20.4699, -0.1906) (-20.5347, -0.1468) knots 0 0 0 1 2 2 2
  spline S129 degree 2 poles (-20.5347, -0.1468) (-20.5914, -0.1095) (-20.7422, -0.0787) (-20.8524, -0.0787) knots 0 0 0 1 2 2 2
  line L254 (-20.8524, -0.0787) -> (-21.1165, -0.0787)
  line L255 (-21.1165, -0.0787) -> (-21.1165, -0.8308)
  line L256 (-21.1165, -0.8308) -> (-20.8832, -0.8308)
  spline S130 degree 2 poles (-20.8832, -0.8308) (-20.7681, -0.8308) (-20.5849, -0.7903) (-20.5217, -0.727) knots 0 0 0 1 2 2 2
  spline S131 degree 2 poles (-20.5217, -0.727) (-20.4634, -0.6719) (-20.4083, -0.5164) (-20.4083, -0.4126) knots 0 0 0 1 2 2 2
  line L257 (-19.8913, -1.8486) -> (-19.217, 0.1514)
  line L258 (-19.217, 0.1514) -> (-18.8896, 0.1514)
  line L259 (-18.8896, 0.1514) -> (-18.2154, -1.8486)
  line L260 (-18.2154, -1.8486) -> (-18.4958, -1.8486)
  line L261 (-18.4958, -1.8486) -> (-18.6773, -1.2894)
  line L262 (-18.6773, -1.2894) -> (-19.4407, -1.2894)
  line L263 (-19.4407, -1.2894) -> (-19.6222, -1.8486)
  line L264 (-19.6222, -1.8486) -> (-19.8913, -1.8486)
  line L265 (-18.7503, -1.0625) -> (-19.0598, -0.1209)
  line L266 (-19.0598, -0.1209) -> (-19.3678, -1.0625)
  line L267 (-19.3678, -1.0625) -> (-18.7503, -1.0625)
  line L268 (-16.867, -1.8486) -> (-18.0258, -1.8486)
  line L269 (-18.0258, -1.8486) -> (-18.0258, 0.1514)
  line L270 (-18.0258, 0.1514) -> (-17.76, 0.1514)
  line L271 (-17.76, 0.1514) -> (-17.76, -1.612)
  line L272 (-17.76, -1.612) -> (-16.867, -1.612)
  line L273 (-16.867, -1.612) -> (-16.867, -1.8486)
  line L274 (-15.961, -1.8486) -> (-16.7357, -1.8486)
  line L275 (-16.7357, -1.8486) -> (-16.7357, -1.6444)
  line L276 (-16.7357, -1.6444) -> (-16.4812, -1.6444)
  line L277 (-16.4812, -1.6444) -> (-16.4812, -0.0528)
  line L278 (-16.4812, -0.0528) -> (-16.7357, -0.0528)
  line L279 (-16.7357, -0.0528) -> (-16.7357, 0.1514)
  line L280 (-16.7357, 0.1514) -> (-15.961, 0.1514)
  line L281 (-15.961, 0.1514) -> (-15.961, -0.0528)
  line L282 (-15.961, -0.0528) -> (-16.2154, -0.0528)
  line L283 (-16.2154, -0.0528) -> (-16.2154, -1.6444)
  line L284 (-16.2154, -1.6444) -> (-15.961, -1.6444)
  line L285 (-15.961, -1.6444) -> (-15.961, -1.8486)
  line L286 (-14.3564, -1.8486) -> (-15.7535, -1.8486)
  line L287 (-15.7535, -1.8486) -> (-15.7535, -1.6006)
  line L288 (-15.7535, -1.6006) -> (-14.6838, -0.0852)
  line L289 (-14.6838, -0.0852) -> (-15.7049, -0.0852)
  line L290 (-15.7049, -0.0852) -> (-15.7049, 0.1514)
  line L291 (-15.7049, 0.1514) -> (-14.384, 0.1514)
  line L292 (-14.384, 0.1514) -> (-14.384, -0.0885)
  line L293 (-14.384, -0.0885) -> (-15.465, -1.612)
  line L294 (-15.465, -1.612) -> (-14.3564, -1.612)
  line L295 (-14.3564, -1.612) -> (-14.3564, -1.8486)
  line L296 (-14.3094, -1.8486) -> (-13.6352, 0.1514)
  line L297 (-13.6352, 0.1514) -> (-13.3078, 0.1514)
  line L298 (-13.3078, 0.1514) -> (-12.6336, -1.8486)
  line L299 (-12.6336, -1.8486) -> (-12.914, -1.8486)
  line L300 (-12.914, -1.8486) -> (-13.0955, -1.2894)
  line L301 (-13.0955, -1.2894) -> (-13.8589, -1.2894)
  line L302 (-13.8589, -1.2894) -> (-14.0404, -1.8486)
  line L303 (-14.0404, -1.8486) -> (-14.3094, -1.8486)
  line L304 (-13.1684, -1.0625) -> (-13.478, -0.1209)
  line L305 (-13.478, -0.1209) -> (-13.7859, -1.0625)
  line L306 (-13.7859, -1.0625) -> (-13.1684, -1.0625)
  spline S132 degree 2 poles (-10.867, -0.8502) (-10.867, -1.1241) (-11.089, -1.565) (-11.2754, -1.6881) knots 0 0 0 1 2 2 2
  spline S133 degree 2 poles (-11.2754, -1.6881) (-11.4277, -1.7838) (-11.7405, -1.8486) (-11.9836, -1.8486) knots 0 0 0 1 2 2 2
  line L307 (-11.9836, -1.8486) -> (-12.4439, -1.8486)
  line L308 (-12.4439, -1.8486) -> (-12.4439, 0.1514)
  line L309 (-12.4439, 0.1514) -> (-11.9885, 0.1514)
  spline S134 degree 2 poles (-11.9885, 0.1514) (-11.7065, 0.1514) (-11.3856, 0.0671) (-11.2721, -0.0074) knots 0 0 0 1 2 2 2
  spline S135 degree 2 poles (-11.2721, -0.0074) (-11.0793, -0.1355) (-10.867, -0.5585) (-10.867, -0.8502) knots 0 0 0 1 2 2 2
  spline S136 degree 2 poles (-11.1441, -0.847) (-11.1441, -0.6168) (-11.2965, -0.2911) (-11.4472, -0.1987) knots 0 0 0 1 2 2 2
  spline S137 degree 2 poles (-11.4472, -0.1987) (-11.5541, -0.1355) (-11.7956, -0.0787) (-11.9755, -0.0787) knots 0 0 0 1 2 2 2
  line L310 (-11.9755, -0.0787) -> (-12.1781, -0.0787)
  line L311 (-12.1781, -0.0787) -> (-12.1781, -1.6185)
  line L312 (-12.1781, -1.6185) -> (-11.9755, -1.6185)
  spline S138 degree 2 poles (-11.9755, -1.6185) (-11.7989, -1.6185) (-11.5315, -1.5617) (-11.4229, -1.4856) knots 0 0 0 1 2 2 2
  spline S139 degree 2 poles (-11.4229, -1.4856) (-11.2835, -1.3916) (-11.1441, -1.0804) (-11.1441, -0.847) knots 0 0 0 1 2 2 2
  spline S140 degree 2 poles (-9.1636, -0.0771) (-9.0501, -0.21) (-8.9237, -0.599) (-8.9237, -0.8486) knots 0 0 0 1 2 2 2
  spline S141 degree 2 poles (-8.9237, -0.8486) (-8.9237, -1.0917) (-9.0469, -1.4856) (-9.1636, -1.6185) knots 0 0 0 1 2 2 2
  spline S142 degree 2 poles (-9.1636, -1.6185) (-9.2867, -1.7578) (-9.6125, -1.8907) (-9.8086, -1.8907) knots 0 0 0 1 2 2 2
  spline S143 degree 2 poles (-9.8086, -1.8907) (-10.0112, -1.8907) (-10.3353, -1.753) (-10.4537, -1.6185) knots 0 0 0 1 2 2 2
  spline S144 degree 2 poles (-10.4537, -1.6185) (-10.5687, -1.4856) (-10.6919, -1.095) (-10.6919, -0.8486) knots 0 0 0 1 2 2 2
  spline S145 degree 2 poles (-10.6919, -0.8486) (-10.6919, -0.5974) (-10.5671, -0.2149) (-10.452, -0.0771) knots 0 0 0 1 2 2 2
  spline S146 degree 2 poles (-10.452, -0.0771) (-10.3353, 0.0558) (-10.0096, 0.1935) (-9.8086, 0.1935) knots 0 0 0 1 2 2 2
  spline S147 degree 2 poles (-9.8086, 0.1935) (-9.6044, 0.1935) (-9.277, 0.0509) (-9.1636, -0.0771) knots 0 0 0 1 2 2 2
  spline S148 degree 2 poles (-9.2008, -0.8486) (-9.2008, -0.6509) (-9.2867, -0.3446) (-9.3645, -0.2441) knots 0 0 0 1 2 2 2
  spline S149 degree 2 poles (-9.3645, -0.2441) (-9.4439, -0.1403) (-9.6676, -0.0366) (-9.807, -0.0366) knots 0 0 0 1 2 2 2
  spline S150 degree 2 poles (-9.807, -0.0366) (-9.9512, -0.0366) (-10.1684, -0.1371) (-10.2511, -0.2441) knots 0 0 0 1 2 2 2
  spline S151 degree 2 poles (-10.2511, -0.2441) (-10.3305, -0.3462) (-10.4148, -0.6541) (-10.4148, -0.8486) knots 0 0 0 1 2 2 2
  spline S152 degree 2 poles (-10.4148, -0.8486) (-10.4148, -1.2424) (-10.0841, -1.6606) (-9.807, -1.6606) knots 0 0 0 1 2 2 2
  spline S153 degree 2 poles (-9.807, -1.6606) (-9.5298, -1.6606) (-9.2008, -1.2424) (-9.2008, -0.8486) knots 0 0 0 1 2 2 2
  spline S154 degree 2 poles (-6.196, -0.8502) (-6.196, -1.1241) (-6.418, -1.565) (-6.6044, -1.6881) knots 0 0 0 1 2 2 2
  spline S155 degree 2 poles (-6.6044, -1.6881) (-6.7567, -1.7838) (-7.0695, -1.8486) (-7.3127, -1.8486) knots 0 0 0 1 2 2 2
  line L313 (-7.3127, -1.8486) -> (-7.773, -1.8486)
  line L314 (-7.773, -1.8486) -> (-7.773, 0.1514)
  line L315 (-7.773, 0.1514) -> (-7.3175, 0.1514)
  spline S156 degree 2 poles (-7.3175, 0.1514) (-7.0355, 0.1514) (-6.7146, 0.0671) (-6.6012, -0.0074) knots 0 0 0 1 2 2 2
  spline S157 degree 2 poles (-6.6012, -0.0074) (-6.4083, -0.1355) (-6.196, -0.5585) (-6.196, -0.8502) knots 0 0 0 1 2 2 2
  spline S158 degree 2 poles (-6.4731, -0.847) (-6.4731, -0.6168) (-6.6255, -0.2911) (-6.7762, -0.1987) knots 0 0 0 1 2 2 2
  spline S159 degree 2 poles (-6.7762, -0.1987) (-6.8832, -0.1355) (-7.1247, -0.0787) (-7.3046, -0.0787) knots 0 0 0 1 2 2 2
  line L316 (-7.3046, -0.0787) -> (-7.5071, -0.0787)
  line L317 (-7.5071, -0.0787) -> (-7.5071, -1.6185)
  line L318 (-7.5071, -1.6185) -> (-7.3046, -1.6185)
  spline S160 degree 2 poles (-7.3046, -1.6185) (-7.1279, -1.6185) (-6.8605, -1.5617) (-6.7519, -1.4856) knots 0 0 0 1 2 2 2
  spline S161 degree 2 poles (-6.7519, -1.4856) (-6.6125, -1.3916) (-6.4731, -1.0804) (-6.4731, -0.847) knots 0 0 0 1 2 2 2
  line L319 (-5.9075, -1.8486) -> (-5.9075, 0.1514)
  line L320 (-5.9075, 0.1514) -> (-4.6563, 0.1514)
  line L321 (-4.6563, 0.1514) -> (-4.6563, -0.0852)
  line L322 (-4.6563, -0.0852) -> (-5.6417, -0.0852)
  line L323 (-5.6417, -0.0852) -> (-5.6417, -0.633)
  line L324 (-5.6417, -0.633) -> (-4.7227, -0.633)
  line L325 (-4.7227, -0.633) -> (-4.7227, -0.8697)
  line L326 (-4.7227, -0.8697) -> (-5.6417, -0.8697)
  line L327 (-5.6417, -0.8697) -> (-5.6417, -1.612)
  line L328 (-5.6417, -1.612) -> (-4.6563, -1.612)
  line L329 (-4.6563, -1.612) -> (-4.6563, -1.8486)
  line L330 (-4.6563, -1.8486) -> (-5.9075, -1.8486)
  line L331 (-1.7908, -1.8486) -> (-2.0566, -1.8486)
  line L332 (-2.0566, -1.8486) -> (-2.0566, -0.1258)
  line L333 (-2.0566, -0.1258) -> (-2.5785, -1.2976)
  line L334 (-2.5785, -1.2976) -> (-2.7405, -1.2976)
  line L335 (-2.7405, -1.2976) -> (-3.2576, -0.1258)
  line L336 (-3.2576, -0.1258) -> (-3.2576, -1.8486)
  line L337 (-3.2576, -1.8486) -> (-3.5055, -1.8486)
  line L338 (-3.5055, -1.8486) -> (-3.5055, 0.1514)
  line L339 (-3.5055, 0.1514) -> (-3.1425, 0.1514)
  line L340 (-3.1425, 0.1514) -> (-2.6433, -0.9621)
  line L341 (-2.6433, -0.9621) -> (-2.1603, 0.1514)
  line L342 (-2.1603, 0.1514) -> (-1.7908, 0.1514)
  line L343 (-1.7908, 0.1514) -> (-1.7908, -1.8486)
  spline S162 degree 2 poles (0.0293, -0.0771) (0.1428, -0.21) (0.2692, -0.599) (0.2692, -0.8486) knots 0 0 0 1 2 2 2
  spline S163 degree 2 poles (0.2692, -0.8486) (0.2692, -1.0917) (0.146, -1.4856) (0.0293, -1.6185) knots 0 0 0 1 2 2 2
  spline S164 degree 2 poles (0.0293, -1.6185) (-0.0939, -1.7578) (-0.4196, -1.8907) (-0.6157, -1.8907) knots 0 0 0 1 2 2 2
  spline S165 degree 2 poles (-0.6157, -1.8907) (-0.8183, -1.8907) (-1.1425, -1.753) (-1.2608, -1.6185) knots 0 0 0 1 2 2 2
  spline S166 degree 2 poles (-1.2608, -1.6185) (-1.3759, -1.4856) (-1.499, -1.095) (-1.499, -0.8486) knots 0 0 0 1 2 2 2
  spline S167 degree 2 poles (-1.499, -0.8486) (-1.499, -0.5974) (-1.3742, -0.2149) (-1.2592, -0.0771) knots 0 0 0 1 2 2 2
  spline S168 degree 2 poles (-1.2592, -0.0771) (-1.1425, 0.0558) (-0.8167, 0.1935) (-0.6157, 0.1935) knots 0 0 0 1 2 2 2
  spline S169 degree 2 poles (-0.6157, 0.1935) (-0.4115, 0.1935) (-0.0841, 0.0509) (0.0293, -0.0771) knots 0 0 0 1 2 2 2
  spline S170 degree 2 poles (-0.008, -0.8486) (-0.008, -0.6509) (-0.0939, -0.3446) (-0.1717, -0.2441) knots 0 0 0 1 2 2 2
  spline S171 degree 2 poles (-0.1717, -0.2441) (-0.2511, -0.1403) (-0.4747, -0.0366) (-0.6141, -0.0366) knots 0 0 0 1 2 2 2
  spline S172 degree 2 poles (-0.6141, -0.0366) (-0.7584, -0.0366) (-0.9755, -0.1371) (-1.0582, -0.2441) knots 0 0 0 1 2 2 2
  spline S173 degree 2 poles (-1.0582, -0.2441) (-1.1376, -0.3462) (-1.2219, -0.6541) (-1.2219, -0.8486) knots 0 0 0 1 2 2 2
  spline S174 degree 2 poles (-1.2219, -0.8486) (-1.2219, -1.2424) (-0.8913, -1.6606) (-0.6141, -1.6606) knots 0 0 0 1 2 2 2
  spline S175 degree 2 poles (-0.6141, -1.6606) (-0.337, -1.6606) (-0.008, -1.2424) (-0.008, -0.8486) knots 0 0 0 1 2 2 2
  line L344 (1.0277, -1.8486) -> (1.0277, -0.0852)
  line L345 (1.0277, -0.0852) -> (0.3567, -0.0852)
  line L346 (0.3567, -0.0852) -> (0.3567, 0.1514)
  line L347 (0.3567, 0.1514) -> (1.9645, 0.1514)
  line L348 (1.9645, 0.1514) -> (1.9645, -0.0852)
  line L349 (1.9645, -0.0852) -> (1.2935, -0.0852)
  line L350 (1.2935, -0.0852) -> (1.2935, -1.8486)
  line L351 (1.2935, -1.8486) -> (1.0277, -1.8486)
  spline S176 degree 2 poles (3.582, -0.0771) (3.6954, -0.21) (3.8219, -0.599) (3.8219, -0.8486) knots 0 0 0 1 2 2 2
  spline S177 degree 2 poles (3.8219, -0.8486) (3.8219, -1.0917) (3.6987, -1.4856) (3.582, -1.6185) knots 0 0 0 1 2 2 2
  spline S178 degree 2 poles (3.582, -1.6185) (3.4588, -1.7578) (3.133, -1.8907) (2.9369, -1.8907) knots 0 0 0 1 2 2 2
  spline S179 degree 2 poles (2.9369, -1.8907) (2.7343, -1.8907) (2.4102, -1.753) (2.2919, -1.6185) knots 0 0 0 1 2 2 2
  spline S180 degree 2 poles (2.2919, -1.6185) (2.1768, -1.4856) (2.0536, -1.095) (2.0536, -0.8486) knots 0 0 0 1 2 2 2
  spline S181 degree 2 poles (2.0536, -0.8486) (2.0536, -0.5974) (2.1784, -0.2149) (2.2935, -0.0771) knots 0 0 0 1 2 2 2
  spline S182 degree 2 poles (2.2935, -0.0771) (2.4102, 0.0558) (2.736, 0.1935) (2.9369, 0.1935) knots 0 0 0 1 2 2 2
  spline S183 degree 2 poles (2.9369, 0.1935) (3.1412, 0.1935) (3.4685, 0.0509) (3.582, -0.0771) knots 0 0 0 1 2 2 2
  spline S184 degree 2 poles (3.5447, -0.8486) (3.5447, -0.6509) (3.4588, -0.3446) (3.381, -0.2441) knots 0 0 0 1 2 2 2
  spline S185 degree 2 poles (3.381, -0.2441) (3.3016, -0.1403) (3.0779, -0.0366) (2.9386, -0.0366) knots 0 0 0 1 2 2 2
  spline S186 degree 2 poles (2.9386, -0.0366) (2.7943, -0.0366) (2.5771, -0.1371) (2.4945, -0.2441) knots 0 0 0 1 2 2 2
  spline S187 degree 2 poles (2.4945, -0.2441) (2.4151, -0.3462) (2.3308, -0.6541) (2.3308, -0.8486) knots 0 0 0 1 2 2 2
  spline S188 degree 2 poles (2.3308, -0.8486) (2.3308, -1.2424) (2.6614, -1.6606) (2.9386, -1.6606) knots 0 0 0 1 2 2 2
  spline S189 degree 2 poles (2.9386, -1.6606) (3.2157, -1.6606) (3.5447, -1.2424) (3.5447, -0.8486) knots 0 0 0 1 2 2 2
  line L352 (5.6614, -1.8486) -> (5.3162, -1.8486)
  line L353 (5.3162, -1.8486) -> (4.6841, -1.0528)
  line L354 (4.6841, -1.0528) -> (4.3794, -1.0528)
  line L355 (4.3794, -1.0528) -> (4.3794, -1.8486)
  line L356 (4.3794, -1.8486) -> (4.1136, -1.8486)
  line L357 (4.1136, -1.8486) -> (4.1136, 0.1514)
  line L358 (4.1136, 0.1514) -> (4.629, 0.1514)
  spline S190 degree 2 poles (4.629, 0.1514) (4.8008, 0.1514) (5.0326, 0.1141) (5.1379, 0.046) knots 0 0 0 1 2 2 2
  spline S191 degree 2 poles (5.1379, 0.046) (5.2433, -0.022) (5.3648, -0.2343) (5.3648, -0.3916) knots 0 0 0 1 2 2 2
  spline S192 degree 2 poles (5.3648, -0.3916) (5.3648, -0.6104) (5.1412, -0.907) (4.9499, -0.9783) knots 0 0 0 1 2 2 2
  line L359 (4.9499, -0.9783) -> (5.6614, -1.8486)
  spline S193 degree 2 poles (5.0877, -0.4126) (5.0877, -0.3251) (5.0261, -0.1906) (4.9612, -0.1468) knots 0 0 0 1 2 2 2
  spline S194 degree 2 poles (4.9612, -0.1468) (4.9045, -0.1095) (4.7538, -0.0787) (4.6436, -0.0787) knots 0 0 0 1 2 2 2
  line L360 (4.6436, -0.0787) -> (4.3794, -0.0787)
  line L361 (4.3794, -0.0787) -> (4.3794, -0.8308)
  line L362 (4.3794, -0.8308) -> (4.6128, -0.8308)
  spline S195 degree 2 poles (4.6128, -0.8308) (4.7279, -0.8308) (4.911, -0.7903) (4.9742, -0.727) knots 0 0 0 1 2 2 2
  spline S196 degree 2 poles (4.9742, -0.727) (5.0326, -0.6719) (5.0877, -0.5164) (5.0877, -0.4126) knots 0 0 0 1 2 2 2
  line L363 (5.8202, -1.8486) -> (5.8202, 0.1514)
  line L364 (5.8202, 0.1514) -> (7.0715, 0.1514)
  line L365 (7.0715, 0.1514) -> (7.0715, -0.0852)
  line L366 (7.0715, -0.0852) -> (6.086, -0.0852)
  line L367 (6.086, -0.0852) -> (6.086, -0.633)
  line L368 (6.086, -0.633) -> (7.005, -0.633)
  line L369 (7.005, -0.633) -> (7.005, -0.8697)
  line L370 (7.005, -0.8697) -> (6.086, -0.8697)
  line L371 (6.086, -0.8697) -> (6.086, -1.612)
  line L372 (6.086, -1.612) -> (7.0715, -1.612)
  line L373 (7.0715, -1.612) -> (7.0715, -1.8486)
  line L374 (7.0715, -1.8486) -> (5.8202, -1.8486)
  spline S197 degree 2 poles (7.9207, -1.8843) (7.7035, -1.8843) (7.3988, -1.7935) (7.2643, -1.7287) knots 0 0 0 1 2 2 2
  line L375 (7.2643, -1.7287) -> (7.2643, -1.3948)
  line L376 (7.2643, -1.3948) -> (7.2838, -1.3948)
  spline S198 degree 2 poles (7.2838, -1.3948) (7.4151, -1.518) (7.7473, -1.6541) (7.9013, -1.6541) knots 0 0 0 1 2 2 2
  spline S199 degree 2 poles (7.9013, -1.6541) (8.1217, -1.6541) (8.347, -1.471) (8.347, -1.3202) knots 0 0 0 1 2 2 2
  spline S200 degree 2 poles (8.347, -1.3202) (8.347, -1.2003) (8.2287, -1.0512) (8.1006, -1.0139) knots 0 0 0 1 2 2 2
  spline S201 degree 2 poles (8.1006, -1.0139) (8.0082, -0.988) (7.8543, -0.9523) (7.7392, -0.9232) knots 0 0 0 1 2 2 2
  spline S202 degree 2 poles (7.7392, -0.9232) (7.6355, -0.8956) (7.4718, -0.8129) (7.4086, -0.7465) knots 0 0 0 1 2 2 2
  spline S203 degree 2 poles (7.4086, -0.7465) (7.347, -0.68) (7.2789, -0.5018) (7.2789, -0.3851) knots 0 0 0 1 2 2 2
  spline S204 degree 2 poles (7.2789, -0.3851) (7.2789, -0.142) (7.6582, 0.1871) (7.9515, 0.1871) knots 0 0 0 1 2 2 2
  spline S205 degree 2 poles (7.9515, 0.1871) (8.1201, 0.1871) (8.4183, 0.1206) (8.5463, 0.0574) knots 0 0 0 1 2 2 2
  line L377 (8.5463, 0.0574) -> (8.5463, -0.2603)
  line L378 (8.5463, -0.2603) -> (8.5269, -0.2603)
  spline S206 degree 2 poles (8.5269, -0.2603) (8.4313, -0.1728) (8.133, -0.0431) (7.9694, -0.0431) knots 0 0 0 1 2 2 2
  spline S207 degree 2 poles (7.9694, -0.0431) (7.7846, -0.0431) (7.5561, -0.2165) (7.5561, -0.3575) knots 0 0 0 1 2 2 2
  spline S208 degree 2 poles (7.5561, -0.3575) (7.5561, -0.4839) (7.6906, -0.6347) (7.817, -0.6687) knots 0 0 0 1 2 2 2
  spline S209 degree 2 poles (7.817, -0.6687) (7.9013, -0.6914) (8.146, -0.7497) (8.227, -0.774) knots 0 0 0 1 2 2 2
  spline S210 degree 2 poles (8.227, -0.774) (8.4329, -0.8373) (8.6241, -1.0917) (8.6241, -1.2781) knots 0 0 0 1 2 2 2
  spline S211 degree 2 poles (8.6241, -1.2781) (8.6241, -1.3964) (8.5285, -1.6233) (8.4426, -1.7027) knots 0 0 0 1 2 2 2
  spline S212 degree 2 poles (8.4426, -1.7027) (8.347, -1.7903) (8.1039, -1.8843) (7.9207, -1.8843) knots 0 0 0 1 2 2 2
  point P0 (0, 0)
  point P1 (-59.7665, -0.8486)
  point P2 (-65.0365, 8.119)
  point P3 (8.6922, -0.8486)
  constraints: 3 midpoint, 4 other
extrude "Extrusão2" add sketch "Esboço2" along normal blind 0.5
